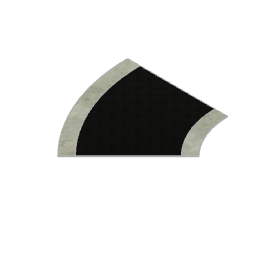
_52 dia 45.cd2838bf-4727-4eac-ac47-c8613db55be0 (Autodesk Fusion 360 design; units mm, degrees)
Autodesk Fusion 360 part; units mm, degrees
sketch "Sketch1" plane through (0, 0, 0) normal (0, 0, 1) x (1, 0, 0)
  circle A0 centre (-662.532, 1929.7788) radius 660.4
  circle A1 centre (-662.532, 1929.7788) radius 1270
  circle A2 centre (-662.532, 1929.7788) radius 558.8
  circle A3 centre (-662.532, 1929.7788) radius 1371.6
  line L0 (-662.532, 1929.7788) -> (-2034.132, 1929.7788)
  line L1 (-662.532, 1929.7788) -> (-1632.3996, 959.9111)
  dimension "d1" = 1320.8
  dimension "d2" = 2540
  dimension "d3" = 1117.6
  dimension "d4" = 2743.2
  dimension "d5" = 135
  constraint concentric A0 A1
  constraint concentric A0 A2
  constraint concentric A1 A3
  constraint coincident A0.centre A1.centre
  constraint coincident A3 L0.end
  constraint horizontal L0
  constraint coincident A3 L1.end
  measures "d1" diameter of A0
  measures "d2" diameter of A1
  measures "d3" diameter of A2
  measures "d4" diameter of A3
  measures "d5" angle of L0 L1
extrude "Extrude1" add sketch "Sketch1" along normal blind 6.35 contours A0 A1 L0 L1 picked at (-1539.6458, 1326.3944)
extrude "Extrude2" add sketch "Sketch1" along normal blind 6.096 contours A0 A2 L0 L1 | A1 A3 L0 L1 picked at (-1285.5885, 1876.7329) picked at (-1996.3539, 1870.1022)
